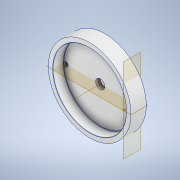
# Autodesk Inventor part: felge
Saved by Autodesk Inventor 2022 (Build 260153000, 153)
## iProperties
Created: 2022-11-16
Part Number: felge
Material: Aluminium 6061
Document SubType Name: Modeling
Designer: Friedrich Walmrath
Density: 2.7 g/cm^3
Appearance: Aluminium - flach
Mass: 30.532 g
Surface Area: 66.7954 cm^2
Volume: 11.3081 cm^3
Author: Friedrich Walmrath
Autodesk Inventor part; units mm, degrees
ref_plane "XY Plane" through (0, 0, 0) normal (0, 0, 1) x (1, 0, 0)
sketch "Skizze1" plane through (0, 0, 0) normal (0, 0, 1) x (1, 0, 0)
  circle A0 centre (0, 0) radius 30
  dimension "d0" = 60
  constraints: 1 centre point, 1 coincident
  measures "d0" diameter of A0
extrude "Extrusion1" add sketch "Skizze1" along normal blind 10
sketch "Skizze2" plane through (0, 0, 10) normal (0, 0, 1) x (1, 0, 0)
  circle A0 centre (0, 0) radius 30 projected
  circle A1 centre (0, 0) radius 24
  circle A2 centre (0, 0) radius 3
  dimension "d3" = 6
  dimension "d4" = 6
  constraints: 2 centre point, 1 coincident
  measures "d3" radial gap between concentric circles of A0 A1
  measures "d4" diameter of A2
extrude "Extrusion2" cut sketch "Skizze2" against normal blind 7 contours A1 | A2
sketch "Skizze3" plane through (0, 0, 10) normal (0, 0, 1) x (1, 0, 0)
  circle A0 centre (0, 0) radius 3
  dimension "d7" = 6
  constraints: 1 centre point, 1 coincident
  measures "d7" diameter of A0
extrude "Extrusion3" cut sketch "Skizze3" along normal through all both and the other way through all
fillet "Rundung1" radius 0.2 1 edges at (-24, 0, 3)
chamfer "Fase1" distance 0.2 angle 45 3 edges at (-30, 0, 0) (-30, 0, 10) (-24, 0, 10)
sketch "Skizze4" plane through (0, 0, 10) normal (0, 0, 1) x (1, 0, 0)
  circle A0 centre (0, 0) radius 27
  circle A1 centre (0, 0) radius 37
  dimension "d14" = 54
  dimension "d15" = 10
  constraints: 2 centre point, 1 coincident
  measures "d14" diameter of A0
  measures "d15" radial gap between concentric circles of A0 A1
extrude "Extrusion4" cut sketch "Skizze4" along normal through all both and the other way through all
ref_plane "Arbeitsebene1" through (22.5, 0, 0) normal (1, 0, 0) x (0, 1, 0)
ref_plane "Arbeitsebene2" through (0, 0, 0) normal (0, 1, 0) x (-1, 0, 0)
hole "Bohrung2" at (22.5, 0, 0) direction (0, 0, 1) diameter 3 depth 3 tip angle 118
pattern_circular "Runde Anordnung2" count 2 over 360 about axis through (0, 0, 10) along (0, 0, 1) of "Bohrung2"
sketch "Skizze6" plane through (0, 0, 10) normal (0, 0, 1) x (1, 0, 0)
  circle A0 centre (-22.5, 0) radius 1.5
  circle A1 centre (0, 0) radius 24.2 projected
  dimension "d25" = 3
  dimension "d26" = 22.5
  constraints: 1 centre point, 1 horizontal alignment
  measures "d25" diameter of A0
  measures "d26" distance of A0.centre A1.centre
sketch "Skizze5" plane through (0, 0, 10) normal (0, 0, 1) x (1, 0, 0)
  circle A0 centre (0, 0) radius 3.2 projected
  circle A1 centre (0, 0) radius 27.5
  circle A2 centre (0, 0) radius 30
  dimension "d18" = 55
  dimension "d19" = 60
  constraints: 2 centre point, 2 coincident
  measures "d18" diameter of A1
  measures "d19" diameter of A2
